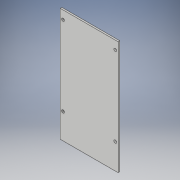
# Autodesk Inventor part: Halterungshauptplatte
Saved by Autodesk Inventor 2019 (Build 230136000, 136)
## iProperties
Created: 2018-09-20
Part Number: Halterungshauptplatte
Material: Generisch
Document SubType Name: Modeling
Designer: nico-
Density: 1 g/cm^3
Appearance: Vorgabe
Author: nico-
Autodesk Inventor part; units mm, degrees
ref_plane "YZ Plane" through (0, 0, 0) normal (1, 0, 0) x (0, 1, 0)
ref_plane "XZ Plane" through (0, 0, 0) normal (0, 1, 0) x (-1, 0, 0)
ref_plane "XY Plane" through (0, 0, 0) normal (0, 0, 1) x (1, 0, 0)
sketch "Skizze1" plane through (0, 0, 0) normal (0, 0, 1) x (1, 0, 0)
  line L0 (50, 85) -> (-52, 85)
  line L1 (-52, 85) -> (-52, -115)
  line L2 (-52, -115) -> (50, -115)
  line L3 (50, -115) -> (50, 85)
  point P0 (0, 0)
  dimension "d0" = 102
  dimension "d1" = 200
  dimension "d10" = 115
  constraints: 8 end point, 2 parallel, 1 horizontal, 1 perpendicular
  measures "d0" distance of L2.end L1.end
  measures "d1" distance of L1.end L0.end
  measures "d10" distance from line of point (0, 0) L2
extrude "Extrusion1" add sketch "Skizze1" along normal blind 3
sketch "Skizze2" plane through (0, 0, 3) normal (0, 0, 1) x (1, 0, 0)
  circle A0 centre (-47, 70) radius 2.5
  circle A1 centre (45, 70) radius 2.5
  circle A2 centre (45, -70) radius 2.5
  circle A3 centre (-47, -70) radius 2.5
  line L0 (50, -115) -> (50, 85) projected
  line L1 (-52, 85) -> (-52, -115) projected
  line L2 (-52, -115) -> (50, -115) projected
  line L3 (50, 85) -> (-52, 85) projected
  point P0 (0, 0)
  dimension "d4" = 5
  dimension "d5" = 5
  dimension "d6" = 5
  dimension "d7" = 5
  dimension "d12" = 5
  dimension "d13" = 5
  dimension "d14" = 45
  dimension "d15" = 45
  dimension "d16" = 5
  dimension "d17" = 5
  dimension "d18" = 15
  dimension "d19" = 15
  constraints: 4 centre point
  measures "d4" diameter of A0
  measures "d5" diameter of A1
  measures "d6" diameter of A2
  measures "d7" diameter of A3
  measures "d12" distance from line of L0 A2.centre
  measures "d13" distance from line of L1 A3.centre
  measures "d14" distance from line of L2 A2.centre
  measures "d15" distance from line of L2 A3.centre
  measures "d16" distance from line of L0 A1.centre
  measures "d17" distance from line of A0.centre L1
  measures "d18" distance from line of L3 A0.centre
  measures "d19" distance from line of L3 A1.centre
extrude "Extrusion2" cut sketch "Skizze2" against normal blind 3 contours A0 | A1 | A2 | A3
